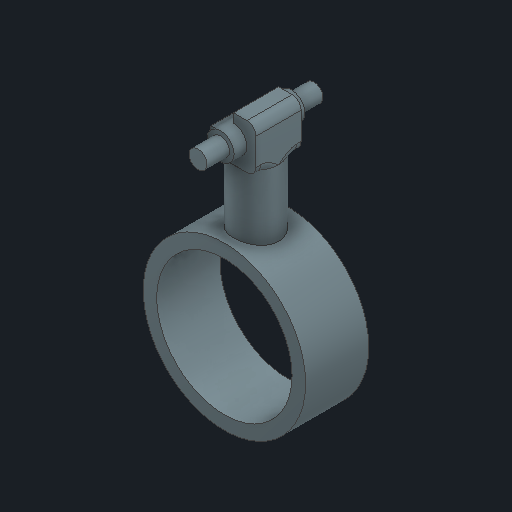
# Autodesk Inventor part: spojka_pol_velke_koleso
Saved by Autodesk Inventor 2022 (Build 260153000, 153)
## iProperties
Created: 2021-12-16
Part Number: spojka_pol_velke_koleso
Material: Generic
Document SubType Name: Modeling
Designer: MatusBarany
Density: 1 g/cm^3
Appearance: Default
Author: MatusBarany
Autodesk Inventor part; units mm, degrees
sketch "Sketch1" plane through (0, 0, 0) normal (0, 0, 1) x (1, 0, 0)
  circle A0 centre (0, 0) radius 18
  circle A1 centre (0, 0) radius 15
  dimension "d0" = 36
  dimension "d1" = 30
  constraints: 2 centre point, 2 coincident
  measures "d0" diameter of A0
  measures "d1" diameter of A1
extrude "Extrusion1" add sketch "Sketch1" along normal blind 14
ref_plane "Work Plane1" through (0, 18, 0) normal (0, 1, 0) x (-1, 0, 0)
sketch "Sketch2" plane through (0, 18, 0) normal (0, 1, 0) x (-1, 0, 0)
  circle A0 centre (0, 7) radius 5
  line L0 (18, 0) -> (-18, 0) projected
  line L1 (18, 14) -> (-18, 14) projected
  point P0 (0, 0)
  dimension "d5" = 7
  dimension "d6" = 14
  dimension "d7" = 10
  constraints: 1 centre point
  measures "d5" distance from line of L0 A0.centre
  measures "d6" distance between parallel lines of L1 L0
  measures "d7" diameter of A0
extrude "Extrusion2" cut sketch "Sketch2" against normal blind 1
sketch "Sketch4" plane through (0, 17, 7) normal (0, 1, 0) x (1, 0, 0)
  circle A0 centre (0, 0) radius 5
  point P0 (0, 7)
  dimension "d10" = 10
  constraints: 1 centre point
  measures "d10" diameter of A0
extrude "Extrusion3" add sketch "Sketch4" along normal blind 20
sketch "Sketch6" plane through (0, 37, 7) normal (0, 1, 0) x (1, 0, 0)
  circle A0 centre (0, 0) radius 5
  line L0 (-18, -7) -> (18, -7) projected
  line L1 (-18, 7) -> (18, 7) projected
  line L2 (0, 7) -> (0, -7)
  point P0 (0, 5)
  point P1 (0, -5)
  dimension "d17" = 7
  dimension "d18" = 14
  dimension "d19" = 10
  constraints: 2 end point, 2 midpoint, 1 centre point
  measures "d17" distance of L2.start A0.centre
  measures "d18" distance between parallel lines of L0 L1
  measures "d19" diameter of A0
extrude "Extrusion4" add sketch "Sketch6" along normal blind 5 contours A0 L2 picked at (1.3031, 1.0391)
ref_plane "Work Plane2" through (5, 17, 7) normal (-1, 0, 0) x (0, 0, 1)
sketch "Sketch9" plane through (0, 37, 2) normal (-1, 0, 0) x (0, 0, 1)
  line L0 (10, 0) -> (0, 0) projected
  line L1 (10, 0) -> (10, 5) projected
  line L2 (0, 5) -> (10, 5) projected
  line L3 (0, 0) -> (0, 5) projected
  point P0 (-2, -37)
extrude "Extrusion6" add sketch "Sketch9" against normal blind 5
sketch "Sketch10" plane through (0, 37, 2) normal (0, -1, 0) x (1, 0, 0)
  arc A0 (5, 5) -> (0, 10) centre (0, 5) ccw projected
  line L0 (5, 10) -> (5, 5) projected
  line L1 (0, 10) -> (5, 10) projected
  arc A1 (0, 0) -> (5, 5) centre (0, 5) ccw projected
  line L2 (0, 0) -> (5, 0) projected
  line L3 (5, 5) -> (5, 0) projected
  point P0 (0, -2)
  point P1 (5, 5)
  point P2 (5, 5)
  point P3 (5, 5)
  point P4 (5, 5)
extrude "Extrusion7" add sketch "Sketch10" along normal blind 5
sketch "Sketch11" plane through (5, 37, 2) normal (1, 0, 0) x (0, 0, -1)
  line L0 (-10, 0) -> (0, 0) projected
  line L1 (0, 5) -> (-10, 5) projected
  line L2 (-10, 5) -> (-10, -5) projected
  line L3 (-5, -5) -> (-10, -5) projected
  line L4 (0, -5) -> (-5, -5) projected
  line L5 (0, 5) -> (0, -5) projected
  point P0 (2, -37)
extrude "Extrusion8" add sketch "Sketch11" against normal blind 10 contours L0 L5 L4 L3 L2
ref_plane "Work Plane3" through (0, 37, 7) normal (0, 0, -1) x (-1, 0, 0)
sketch "Sketch13" plane through (0, 37, 7) normal (0, 0, -1) x (-1, 0, 0)
  line L0 (-5, 5) -> (-5, -5) projected
  line L1 (0, 5) -> (-5, 5) projected
  line L2 (0, 0) -> (0, 5) projected
  line L3 (0, 0) -> (5, 0) projected
  line L4 (5, -5) -> (5, 0) projected
  line L5 (0, -5) -> (5, -5) projected
  line L6 (-5, -5) -> (0, -5) projected
  line L7 (0, 0) -> (5, 0) projected
  circle A0 centre (0, 0) radius 3
  point P0 (0, -37)
  dimension "d47" = 6
  constraints: 1 centre point, 1 coincident
  measures "d47" diameter of A0
extrude "Extrusion10" add sketch "Sketch13" along normal mid plane 15.7143 contours A0 L3 L2 | L2 L3 A0
sketch "Sketch14" plane through (0, 37, -0.8571) normal (0, 0, -1) x (-1, 0, 0)
  circle A0 centre (0, 0) radius 3 projected
  circle A1 centre (0, 0) radius 2
  point P0 (0, -37)
  dimension "d50" = 4
  constraints: 1 centre point, 1 coincident
  measures "d50" diameter of A1
extrude "Extrusion11" add sketch "Sketch14" along normal blind 5 and the other way blind 20.7143 contours A1
fillet "Fillet1" radius 2 5 edges at (-5, 32, 9.5) (-5, 32, 4.5) (5, 32, 9.5) (5, 32, 4.5) (5, 42, 7)
equation "\"d5\" = 0.5 * d6"
equation "\"d17\" = 0.5 * d18"
body "Solid1"
